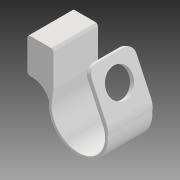
# Autodesk Inventor part: ValveSpring
Saved by Autodesk Inventor 2020 (Build 240168000, 168)
## iProperties
Created: 2021-02-05
Part Number: ValveSpring
Material: Generic
Document SubType Name: Modeling
Designer: DDeGo
Density: 1 g/cm^3
Appearance: Default
Author: DDeGo
Autodesk Inventor part; units mm, degrees
ref_plane "YZ Plane" through (0, 0, 0) normal (1, 0, 0) x (0, 1, 0)
ref_plane "XZ Plane" through (0, 0, 0) normal (0, 1, 0) x (-1, 0, 0)
ref_plane "XY Plane" through (0, 0, 0) normal (0, 0, 1) x (1, 0, 0)
sketch "Sketch1" plane through (0, 0, 0) normal (0, 0, 1) x (1, 0, 0)
  line L0 (-0.85, -1.35) -> (0.85, -1.35)
  line L1 (0.85, -1.35) -> (0.85, 1.35)
  line L2 (0.85, 1.35) -> (-0.85, 1.35)
  line L3 (-0.85, 1.35) -> (-0.85, -1.35)
  line L4 (-0.85, -1.35) -> (0.85, 1.35) construction
  line L5 (0.85, -1.35) -> (-0.85, 1.35) construction
  line L6 (7.1105, -2.8923) -> (4.8846, 1.881)
  line L7 (4.8846, 1.881) -> (5.3378, 2.0923)
  line L8 (5.3378, 2.0923) -> (7.6622, -2.8923)
  line L9 (-1.45, 1.95) -> (1.45, 1.95)
  line L10 (1.45, 1.95) -> (1.45, -1.95)
  line L11 (1.148, -1.95) -> (-1.45, -1.95)
  line L12 (-1.45, -1.95) -> (-1.45, 1.95)
  line L13 (1.45, -1.95) -> (1.148, -1.95) construction
  line L14 (1.148, -1.95) -> (0.9806, -3.3133)
  line L15 (0.9806, -3.3133) -> (1.2826, -3.3133) construction
  line L16 (1.2826, -3.3133) -> (1.45, -1.95)
  line L17 (7.6622, -2.8923) -> (7.1105, -2.8923) construction
  line L18 (7.2357, -3.3923) -> (7.537, -3.3923) construction
  arc A0 (1.2826, -3.3133) -> (7.2357, -3.3923) centre (4.2548, -3.6783) ccw
  arc A1 (0.9806, -3.3133) -> (7.537, -3.3923) centre (4.2548, -3.6783) ccw
  line L19 (7.537, -3.3923) -> (7.6622, -2.8923)
  line L20 (7.1105, -2.8923) -> (7.2357, -3.3923)
  point P0 (0, 0)
  point P1 (6.5, -0.4)
  dimension "d0" = 1.7
  dimension "d1" = 2.7
  dimension "d4" = 0.5
  dimension "d5" = 5.5
  dimension "d16" = 0.6
  dimension "d17" = 0.6
  dimension "d18" = 0.6
  dimension "d19" = 0.6
  dimension "d20" = 25
  dimension "d21" = 6.5
  dimension "d22" = 0.3
  dimension "d25" = 0.5
  dimension "d38" = 83
  dimension "d39" = 0.4
  constraints: 43 end point, 7 parallel, 5 point on circle, 4 horizontal, 4 perpendicular, 3 midpoint, 2 centre point, 1 coincident, 1 equal length, 1 tangent
  measures "d0" distance of L1.end L2.end
  measures "d1" distance of L0.end L1.end
  measures "d4" distance between parallel lines of L8 L6
  measures "d5" distance of L8.end L7.end
  measures "d16" distance between parallel lines of L9 L2
  measures "d17" distance between parallel lines of L12 L3
  measures "d18" distance between parallel lines of L11 L0
  measures "d19" distance between parallel lines of L1 L10
  measures "d20" angle of L6 L10
  measures "d21" horizontal distance of point (0, 0) point (6.5, -0.4)
  measures "d22" radial gap between concentric circles of A1 A0
  measures "d25" distance between parallel lines of L17 L18
  measures "d38" angle of L11 L14
  measures "d39" vertical distance of point (0, 0) point (6.5, -0.4)
extrude "Extrusion1" add sketch "Sketch1" along normal blind 5
fillet "Fillet1" radius 2 5 edges at (1.148, -1.95, 2.5) (7.537, -3.3923, 2.5) (7.6622, -2.8923, 2.5) (7.1105, -2.8923, 2.5) (7.2357, -3.3923, 2.5)
fillet "Fillet1" radius 0.3 3 edges at (-1.45, -1.95, 2.5) (-1.45, 1.95, 2.5) (1.45, 1.95, 2.5)
sketch "Sketch3" plane through (0, 0, 5) normal (0, 0, 1) x (1, 0, 0)
  line L0 (-0.85, 1.35) -> (0.85, 1.35) projected
  line L1 (-0.85, -1.35) -> (-0.85, 1.35) projected
  line L2 (0.85, 1.35) -> (0.85, -1.35) projected
  line L3 (0.85, -1.35) -> (-0.85, -1.35) projected
  point P0 (0, 0)
extrude "Extrusion3" add sketch "Sketch3" against normal blind 1
sketch "Sketch4" plane through (5.3378, 2.0923, 5) normal (0.9063078, 0.4226183, 0) x (0, 0, -1)
  line L0 (0, -4.8077) -> (5, 0) construction
  circle A0 centre (2.5, -2.4038) radius 1.5
  line L1 (0, -4.8077) -> (0, 0) projected
  line L2 (5, -4.8077) -> (5, 0) projected
  dimension "d33" = 3
  constraints: 2 end point, 1 centre point, 1 midpoint
  measures "d33" diameter of A0
extrude "Extrusion4" cut sketch "Sketch4" against normal up to surface (0.5 mm away)
fillet "Fillet3" radius 1 2 edges at (5.1112, 1.9867, 0) (5.1112, 1.9867, 5)
body "Solid1"
